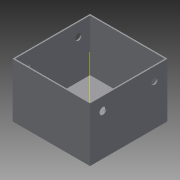
# Autodesk Inventor part: locomotion box
Saved by Autodesk Inventor 2015 (Build 190159000, 159)
## iProperties
Created: 2014-10-11
Part Number: locomotion box
Material: Generic
Document SubType Name: Modeling
Designer: ericd_000
Density: 1 g/cm^3
Appearance: Default
Author: ericd_000
Autodesk Inventor part; units mm, degrees
ref_plane "YZ Plane" through (0, 0, 0) normal (1, 0, 0) x (0, 1, 0)
ref_plane "XZ Plane" through (0, 0, 0) normal (0, 1, 0) x (-1, 0, 0)
ref_plane "XY Plane" through (0, 0, 0) normal (0, 0, 1) x (1, 0, 0)
sketch "Sketch1" plane through (0, 0, 0) normal (0, 0, 1) x (1, 0, 0)
  line L0 (-150, 150) -> (150, 150)
  line L1 (150, 150) -> (150, -150)
  line L2 (150, -150) -> (-150, -150)
  line L3 (-150, -150) -> (-150, 150)
  point P0 (0, 0)
  point P1 (150, 0)
  point P2 (0, 150)
  dimension "d0" = 300
  dimension "d1" = 300
  constraints: 8 end point, 2 midpoint, 2 parallel, 1 horizontal, 1 horizontal alignment, 1 perpendicular, 1 vertical alignment
  measures "d0" distance of L0.start L0.end
  measures "d1" distance of L0.end L1.end
extrude "Extrusion1" add sketch "Sketch1" along normal blind 10
sketch "Sketch2" plane through (0, 0, 10) normal (0, 0, 1) x (1, 0, 0)
  line L0 (-150, 150) -> (150, 150)
  line L1 (150, 150) -> (150, -150)
  line L2 (150, -150) -> (-150, -150)
  line L3 (-150, -150) -> (-150, 150)
  line L4 (145, 145) -> (-145, 145)
  line L5 (-145, 145) -> (-145, -145)
  line L6 (-145, -145) -> (145, -145)
  line L7 (145, -145) -> (145, 145)
  point P0 (0, 0)
  dimension "d4" = 5
  constraints: 16 end point, 4 parallel, 2 perpendicular, 1 horizontal, 3 other
  measures "d4" distance between parallel lines of L3 L5
extrude "Extrusion2" add sketch "Sketch2" along normal blind 200
sketch "Sketch3" plane through (-150, -150, 0) normal (-1, 0, 0) x (0, 0, 1)
  circle A0 centre (160, 250) radius 12.5
  circle A1 centre (160, 50) radius 13.3073
  line L0 (0, 300) -> (210, 300) projected
  line L1 (0, 0) -> (210, 0) projected
  line L2 (210, 300) -> (210, 0) projected
  point P0 (0, 150)
  dimension "d7" = 25
  dimension "d8" = 50
  dimension "d9" = 50
  dimension "d10" = 50
  dimension "d11" = 50
  constraints: 2 centre point
  measures "d7" diameter of A0
  measures "d8" distance from line of L0 A0.centre
  measures "d9" distance from line of L1 A1.centre
  measures "d10" distance from line of L2 A1.centre
  measures "d11" distance from line of L2 A0.centre
extrude "Extrusion3" cut sketch "Sketch3" against normal up to surface (5 mm away)
mirror "Mirror1" about plane through (0, 0, 0) normal (1, 0, 0) of "Extrusion3"
sketch "Sketch6" plane through (0, 0, 0) normal (0, 0, -1) x (-1, 0, 0)
  circle A0 centre (0, 0) radius 59.25
  dimension "d21" = 118.5
  constraints: 1 centre point, 1 coincident
  measures "d21" diameter of A0
extrude "Extrusion6" cut sketch "Sketch6" against normal blind 5
sketch "Sketch7" plane through (0, 0, 5) normal (0, 0, -1) x (-1, 0, 0)
  circle A0 centre (42.997, -32.6689) radius 2
  line L0 (42.997, -32.6689) -> (0, 0) construction
  dimension "d24" = 54
  dimension "d25" = 4
  constraints: 2 end point, 1 centre point
  measures "d24" distance of L0.start L0.end
  measures "d25" diameter of A0
extrude "Extrusion7" cut sketch "Sketch7" against normal up to surface (5 mm away)
pattern_circular "Circular Pattern1" count 10 over 360 about axis through (0, 0, 5) along (0, 0, 1) of "Extrusion7"
body "Solid1"
